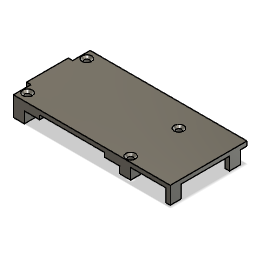
case_lid (Autodesk Fusion 360 design; units mm, degrees)
Autodesk Fusion 360 part; units mm, degrees
note: some values were not read from the file. Set by a fixed rule: which sketch regions a step uses.
sketch "Sketch1" plane through (0, 0, 0) normal (0, 1, 0) x (1, 0, 0)
  line L0 (0, 0) -> (71.7, 0)
  line L1 (71.7, 0) -> (71.7, -35.1)
  line L2 (71.7, -35.1) -> (0, -35.1)
  line L3 (0, -35.1) -> (0, -27.1)
  line L4 (0, -27.1) -> (-2, -27.1)
  line L5 (-2, -27.1) -> (-2, -8)
  line L6 (-2, -8) -> (0, -8)
  line L7 (0, -8) -> (0, 0)
  dimension "d1" = 71.7
  dimension "d2" = 35.1
  dimension "d32" = 8
  dimension "d33" = 8
  dimension "d34" = 2
  dimension "d35" = 2
  constraint horizontal L0
  constraint vertical L1
  constraint horizontal L2
  constraint coincident L0.start L7.end
  constraint perpendicular L2 L3
  constraint perpendicular L3 L4
  constraint perpendicular L4 L5
  constraint perpendicular L5 L6
  constraint perpendicular L0 L7
  measures "d1" distance of L0.start L0.end
  measures "d2" distance of L0.start L2.end
  measures "d32" distance of L2.end L3.end
  measures "d33" distance of L6.end L0.start
  measures "d34" distance of L5.end L6.end
  measures "d35" distance of L3.end L4.end
extrude "Extrude1" add sketch "Sketch1" along normal blind 2
sketch "Sketch2" plane through (0, 0, 0) normal (0, -1, 0) x (1, 0, 0)
  line L0 (71.7, 35.1) -> (0, 35.1)
  line L1 (0, 0) -> (71.7, 0)
  line L2 (71.7, 0) -> (71.7, 35.1)
  line L3 (0, 35.1) -> (5, 35.1)
  line L4 (5, 35.1) -> (5, 27.1)
  line L5 (5, 27.1) -> (0, 27.1)
  line L6 (0, 27.1) -> (0, 35.1)
  line L7 (0, 0) -> (5, 0)
  line L8 (5, 0) -> (5, 8)
  line L9 (5, 8) -> (0, 8)
  line L10 (0, 8) -> (0, 0)
  line L11 (-2, 8) -> (0, 8)
  line L12 (0, 8) -> (0, 0)
  line L13 (0, 35.1) -> (0, 27.1)
  line L14 (0, 27.1) -> (-2, 27.1)
  line L15 (-2, 27.1) -> (-2, 8)
  dimension "d5" = 5
  dimension "d6" = 8
  dimension "d7" = 8
  dimension "d8" = 5
  constraint horizontal L3
  constraint vertical L4
  constraint horizontal L5
  constraint vertical L6
  constraint coincident L0.end L3.start
  constraint horizontal L7
  constraint vertical L8
  constraint horizontal L9
  constraint vertical L10
  constraint coincident L1.start L7.start
  measures "d5" distance of L0.end L3.end
  measures "d6" distance of L0.end L5.end
  measures "d7" distance of L1.start L9.end
  measures "d8" distance of L8.end L9.end
extrude "Extrude2" add sketch "Sketch2" along normal blind 7 contours L0 L3 L4 L5 L6 L13 | L1 L7 L8 L9 L10 L12
sketch "Sketch3" plane through (0, 0, 0) normal (0, -1, 0) x (1, 0, 0)
  line L0 (5, 8) -> (5, 0)
  line L1 (5, 0) -> (71.7, 0)
  line L2 (71.7, 0) -> (71.7, 35.1)
  line L3 (71.7, 35.1) -> (5, 35.1)
  line L4 (5, 35.1) -> (5, 27.1)
  line L5 (5, 27.1) -> (0, 27.1)
  line L6 (0, 8) -> (5, 8)
  line L7 (48.6, 35.1) -> (53.6, 35.1)
  line L8 (53.6, 35.1) -> (53.6, 30.1)
  line L9 (53.6, 30.1) -> (48.6, 30.1)
  line L10 (48.6, 30.1) -> (48.6, 35.1)
  line L11 (48.6, 13) -> (53.6, 13)
  line L12 (53.6, 13) -> (53.6, 8)
  line L13 (53.6, 8) -> (48.6, 8)
  line L14 (48.6, 8) -> (48.6, 13)
  line L15 (0, 27.1) -> (-2, 27.1)
  line L16 (-2, 27.1) -> (-2, 8)
  line L17 (-2, 8) -> (0, 8)
  dimension "d17" = 5
  dimension "d18" = 5
  dimension "d20" = 18.1
  dimension "d21" = 5
  dimension "d22" = 5
  dimension "d31" = 8
  constraint horizontal L7
  constraint vertical L8
  constraint horizontal L9
  constraint vertical L10
  constraint horizontal L11
  constraint vertical L12
  constraint horizontal L13
  constraint vertical L14
  constraint collinear L8 L12
  constraint coincident L3 L7.end
  measures "d17" distance of L7.start L7.end
  measures "d18" distance of L7.end L8.end
  measures "d20" distance of L2 L8
  measures "d21" distance of L11.start L13.end
  measures "d22" distance of L11.start L11.end
  measures "d31" distance of L1 L13
extrude "Extrude3" add sketch "Sketch3" along normal blind 5 contours L3 L7 L8 L9 L10 | L11 L12 L13 L14
sketch "Sketch4" plane through (0, 2, 0) normal (0, 1, 0) x (-1, 0, 0)
  line L0 (0, 8) -> (2, 8)
  line L1 (2, 8) -> (2, 27.1)
  line L2 (2, 27.1) -> (0, 27.1)
  line L3 (0, 27.1) -> (0, 35.1)
  line L4 (0, 35.1) -> (-71.7, 35.1)
  line L5 (-71.7, 35.1) -> (-71.7, 0)
  line L6 (-71.7, 0) -> (0, 0)
  line L7 (0, 0) -> (0, 8)
  line L8 (-5, 27.1) -> (-5, 35.1)
  line L9 (2, 17.55) -> (-71.7, 17.55)
  line L10 (-53.6, 30.1) -> (-53.6, 35.1)
  line L11 (-53.6, 13) -> (-48.6, 13)
  line L12 (-48.6, 13) -> (-48.6, 8)
  point P0 (-2.5, 31.1)
  point P1 (-51.1, 32.6)
  point P2 (-2.5, 4)
  point P3 (-51.1, 10.5)
  dimension "d36" = 4
  dimension "d37" = 2.5
  dimension "d38" = 2.5
  dimension "d39" = 2.5
  dimension "d40" = 2.5
  dimension "d41" = 2.5
  constraint midpoint L1 L9.start
  constraint midpoint L5 L9.end
  constraint symmetric P0 L9 P2
  measures "d36" distance of L4 P0
  measures "d37" distance of P0 L8
  measures "d38" distance of L4 P1
  measures "d39" distance of P1 L10
  measures "d40" distance of P3 L11
  measures "d41" distance of P3 L12
hole "Hole5" at (2.5, 2, 4) at (2.5, 2, 31.1) at (51.1, 2, 10.5) at (51.1, 2, 32.6) direction (0, -1, 0) diameter 2.4 depth 9 tip angle 118 countersink diameter 4.4 countersink angle 90
sketch "Sketch5" plane through (0, 0, 0) normal (0, -1, 0) x (1, 0, 0)
  line L0 (48.6, 8) -> (48.6, 13)
  line L1 (48.6, 13) -> (53.6, 13)
  line L2 (53.6, 13) -> (53.6, 8)
  line L3 (53.6, 8) -> (48.6, 8)
  line L4 (53.6, 35.1) -> (53.6, 30.1)
  line L5 (53.6, 30.1) -> (48.6, 30.1)
  line L6 (48.6, 30.1) -> (48.6, 35.1)
  line L7 (48.6, 35.1) -> (5, 35.1)
  line L8 (5, 35.1) -> (5, 27.1)
  line L9 (5, 27.1) -> (0, 27.1)
  line L10 (0, 27.1) -> (-2, 27.1)
  line L11 (-2, 27.1) -> (-2, 8)
  line L12 (-2, 8) -> (0, 8)
  line L13 (0, 8) -> (5, 8)
  line L14 (5, 8) -> (5, 0)
  line L15 (5, 0) -> (71.7, 0)
  line L16 (71.7, 0) -> (71.7, 35.1)
  line L17 (71.7, 35.1) -> (53.6, 35.1)
  line L18 (53.6, 13) -> (55.6, 13)
  line L19 (55.6, 13) -> (55.6, 8)
  line L20 (55.6, 8) -> (53.6, 8)
  line L21 (53.6, 8) -> (53.6, 13)
  line L22 (71.7, 8) -> (69.7, 8)
  line L23 (69.7, 8) -> (69.7, 3)
  line L24 (69.7, 3) -> (71.7, 3)
  line L25 (71.7, 3) -> (71.7, 8)
  line L26 (71.7, 35.1) -> (69.7, 35.1)
  line L27 (69.7, 35.1) -> (69.7, 30.1)
  line L28 (69.7, 30.1) -> (71.7, 30.1)
  line L29 (71.7, 30.1) -> (71.7, 35.1)
  dimension "d47" = 2
  dimension "d48" = 2
  dimension "d49" = 5
  constraint horizontal L18
  constraint vertical L19
  constraint horizontal L20
  constraint vertical L21
  constraint coincident L1.end L2.start
  constraint collinear L3 L20
  constraint horizontal L22
  constraint vertical L23
  constraint horizontal L24
  constraint vertical L25
  constraint coincident L16 L22.start
  constraint collinear L20 L22
  constraint horizontal L26
  constraint vertical L27
  constraint horizontal L28
  constraint vertical L29
  constraint coincident L16.end L17.start
  constraint collinear L23 L27
  constraint collinear L5 L28
  measures "d47" distance of L19.end L2.end
  measures "d48" distance of L23.end L24.end
  measures "d49" distance of L22.end L23.end
extrude "Extrude4" add sketch "Sketch5" along normal blind 5.9 contours L2 L18 L19 L20 L21 | L16 L17 L26 L27 L28 L29 | L16 L22 L23 L24 L25
sketch "Sketch6" plane through (0, 0, 0) normal (0, -1, 0) x (1, 0, 0)
  line L0 (69.7, 30.1) -> (69.7, 35.1)
  line L1 (69.7, 35.1) -> (53.6, 35.1)
  line L2 (53.6, 35.1) -> (53.6, 30.1)
  line L3 (53.6, 30.1) -> (48.6, 30.1)
  line L4 (48.6, 30.1) -> (48.6, 35.1)
  line L5 (48.6, 35.1) -> (5, 35.1)
  line L6 (5, 35.1) -> (5, 27.1)
  line L7 (5, 27.1) -> (0, 27.1)
  line L8 (0, 27.1) -> (-2, 27.1)
  line L9 (-2, 27.1) -> (-2, 8)
  line L10 (-2, 8) -> (0, 8)
  line L11 (0, 8) -> (5, 8)
  line L12 (5, 8) -> (5, 0)
  line L13 (5, 0) -> (71.7, 0)
  line L14 (71.7, 0) -> (71.7, 3)
  line L15 (71.7, 3) -> (69.7, 3)
  line L16 (69.7, 3) -> (69.7, 8)
  line L17 (69.7, 8) -> (71.7, 8)
  line L18 (71.7, 8) -> (71.7, 30.1)
  line L19 (71.7, 30.1) -> (69.7, 30.1)
  line L20 (48.6, 13) -> (55.6, 13)
  line L21 (55.6, 13) -> (55.6, 8)
  line L22 (55.6, 8) -> (48.6, 8)
  line L23 (48.6, 8) -> (48.6, 13)
  line L24 (5, 35.1) -> (12, 35.1)
  line L25 (12, 35.1) -> (12, 27.1)
  line L26 (12, 27.1) -> (5, 27.1)
  line L27 (5, 27.1) -> (5, 35.1)
  line L28 (5, 8) -> (12, 8)
  line L29 (12, 8) -> (12, 0)
  line L30 (12, 0) -> (5, 0)
  line L31 (5, 0) -> (5, 8)
  line L32 (48.6, 35.1) -> (41.6, 35.1)
  line L33 (41.6, 35.1) -> (41.6, 30.1)
  line L34 (41.6, 30.1) -> (48.6, 30.1)
  line L35 (48.6, 30.1) -> (48.6, 35.1)
  line L36 (48.6, 13) -> (41.6, 13)
  line L37 (41.6, 13) -> (41.6, 8)
  line L38 (41.6, 8) -> (48.6, 8)
  line L39 (48.6, 8) -> (48.6, 13)
  dimension "d52" = 7
  dimension "d53" = 7
  constraint horizontal L24
  constraint vertical L25
  constraint horizontal L26
  constraint vertical L27
  constraint coincident L5.end L6.start
  constraint collinear L7 L26
  constraint horizontal L28
  constraint vertical L29
  constraint horizontal L30
  constraint vertical L31
  constraint coincident L13 L29.end
  constraint coincident L11.end L12.start
  constraint collinear L25 L29
  constraint horizontal L32
  constraint vertical L33
  constraint horizontal L34
  constraint vertical L35
  constraint coincident L4.end L5.start
  constraint collinear L3 L34
  constraint horizontal L36
  constraint vertical L37
  constraint horizontal L38
  constraint vertical L39
  constraint coincident L20.start L23.end
  constraint collinear L22 L38
  constraint collinear L33 L37
  measures "d52" distance of L5.end L24.end
  measures "d53" distance of L4.end L32.end
extrude "Extrude5" add sketch "Sketch6" along normal blind 1.9 contours L4 L5 L32 L33 L34 L35 | L5 L6 L24 L25 L26 L27 | L12 L13 L28 L29 L30 L31 | L23 L36 L37 L38 L39
